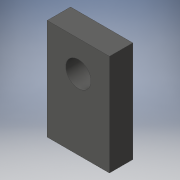
# Autodesk Inventor part: OmniSupportFront
Saved by Autodesk Inventor 2016 (Build 200138000, 138)
## iProperties
Created: 2016-12-02
Part Number: OmniSupportFront
Material: Generic
Document SubType Name: Modeling
Designer: Evan Phil George
Density: 1 g/cm^3
Appearance: Default
Author: Evan Phil George
Autodesk Inventor part; units mm, degrees
ref_plane "YZ Plane" through (0, 0, 0) normal (1, 0, 0) x (0, 1, 0)
ref_plane "XZ Plane" through (0, 0, 0) normal (0, 1, 0) x (-1, 0, 0)
ref_plane "XY Plane" through (0, 0, 0) normal (0, 0, 1) x (1, 0, 0)
sketch "Sketch1" plane through (0, 0, 0) normal (0, 1, 0) x (-1, 0, 0)
  line L0 (20, -7.5) -> (-20, -7.5)
  line L1 (-20, -7.5) -> (-20, 7.5)
  line L2 (-20, 7.5) -> (20, 7.5)
  line L3 (20, 7.5) -> (20, -7.5)
  point P0 (0, 0)
  dimension "d0" = 40
  dimension "d1" = 15
  dimension "d2" = 7.5
  dimension "d3" = 20
  constraints: 8 end point, 2 parallel, 1 horizontal, 1 perpendicular
  measures "d0" distance of L0.start L0.end
  measures "d1" distance of L0.end L1.end
  measures "d2" distance from line of point (0, 0) L0
  measures "d3" distance from line of point (0, 0) L3
extrude "Extrusion1" add sketch "Sketch1" along normal blind 65
sketch "Sketch2" plane through (0, 0, 0) normal (0, -1, 0) x (1, 0, 0)
  line L0 (0, 0) -> (0, 0.5)
  line L1 (0, 0.5) -> (8, 0.5)
  line L2 (0, 0.5) -> (-8, 0.5)
  circle A0 centre (-8, 0.5) radius 1.925
  circle A1 centre (8, 0.5) radius 1.925
  dimension "d21" = 0.5
  dimension "d22" = 8
  dimension "d23" = 8
  dimension "d24" = 3.85
  dimension "d25" = 3.85
  constraints: 6 end point, 2 centre point, 2 coincident, 1 horizontal, 1 perpendicular, 1 vertical
  measures "d21" distance of L0.start L0.end
  measures "d22" distance of L0.end L1.end
  measures "d23" distance of L0.end L2.end
  measures "d24" diameter of A0
  measures "d25" diameter of A1
extrude "Extrusion2" cut sketch "Sketch2" against normal blind 13.7
sketch "Sketch3" plane through (-20, 0, 7.5) normal (0, 0, 1) x (1, 0, 0)
  line L0 (20, 0) -> (20, 45.2)
  circle A0 centre (20, 45.2) radius 8.125
  dimension "d12" = 45.2
  dimension "d13" = 16.25
  constraints: 2 end point, 1 centre point, 1 coincident, 1 vertical
  measures "d12" distance of L0.start L0.end
  measures "d13" diameter of A0
extrude "Extrusion3" cut sketch "Sketch3" against normal blind 20
body "Solid1"
